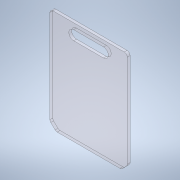
# Autodesk Inventor part: J010355
Saved by Autodesk Inventor 2020.3 (Build 243373000, 373)
## iProperties
RuleStatus: InUse
AfterDocSave0: file://Part Number Cleaner
Created: 2022-05-24
Material: ACRYLIC, CLEAR
Catalog Web Link: https://www.janelia.org/
Vendor: HHMI: JRC - jET
Document SubType Name: Modeling
Designer: arnoldj
Density: 0.66 g/cm^3
Appearance: Polycarbonate (Clear)
Part Number: J010355
Project: COMMON
Description: FB BTM PLATE
LAB/DEPT: COMMON
REQUESTING SCIENTIST: COMMON
SURFACE ROUGHNESS: N/A
DESIGN DEPARTMENT: COMMON
SPECIAL FINISH: NONE
ALTERED ITEM PART NUMBER: N/A
ALTERED ITEM VENDOR: N/A
ALTERED ITEM DESCRIPTION: N/A
Title: Standard
Author: arnoldj
Revision Number: 0
Autodesk Inventor part; units mm, degrees
ref_plane "YZ Plane" through (0, 0, 0) normal (1, 0, 0) x (0, 1, 0)
ref_plane "XZ Plane" through (0, 0, 0) normal (0, 1, 0) x (-1, 0, 0)
ref_plane "XY Plane" through (0, 0, 0) normal (0, 0, 1) x (1, 0, 0)
sketch "Sketch1" plane through (0, 0, 0) normal (0, 0, 1) x (1, 0, 0)
  line L0 (0, 76.454) -> (0, -76.454) projected
  line L1 (-57.4294, 0) -> (57.4294, 0) projected
  line L2 (41.021, -54.61) -> (-41.021, -54.61)
  line L3 (-41.021, -54.61) -> (-41.021, 54.61)
  line L4 (-41.021, 54.61) -> (41.021, 54.61)
  line L5 (41.021, 54.61) -> (41.021, -54.61)
  line L6 (41.021, -54.61) -> (-41.021, 54.61) construction
  line L7 (-41.021, -54.61) -> (41.021, 54.61) construction
  line L8 (15.875, 43.18) -> (-15.875, 43.18) construction
  line L9 (15.875, 48.26) -> (-15.875, 48.26)
  line L10 (-15.875, 38.1) -> (15.875, 38.1)
  arc A0 (15.875, 38.1) -> (15.875, 48.26) centre (15.875, 43.18) ccw
  arc A1 (-15.875, 48.26) -> (-15.875, 38.1) centre (-15.875, 43.18) ccw
  point P0 (0, 0)
  point P1 (0, 43.18)
  dimension "d0" = 82.042
  dimension "d1" = 109.22
  dimension "d4" = 31.75
  dimension "d5" = 6.35
  dimension "d6" = 5.08
  constraints: 20 end point, 4 point on circle, 4 tangent, 3 midpoint, 3 parallel, 2 centre point, 2 perpendicular, 1 horizontal, 1 point on line
  measures "d0" distance of L3.end L4.end
  measures "d1" distance of L2.end L3.end
  measures "d4" distance of L9.start L9.end
  measures "d5" distance between parallel lines of L4 L9
  measures "d6" radius of A1
extrude "Extrusion1" add sketch "Sketch1" along normal blind 2.9972 contours L4 L5 L1 L0 L10 A0 L9 | L0 L9 A1 L10 L1 L3 L4 | L1 L0 L2 L3 | L5 L2 L0 L1
fillet "Fillet1" radius 3.175 2 edges at (-41.021, 54.61, 1.4986) (41.021, 54.61, 1.4986)
chamfer "Chamfer1" distance 6.35 angle 45 2 edges at (41.021, -54.61, 1.4986) (-41.021, -54.61, 1.4986)
fillet "Fillet2" radius 3.175 4 edges at (-41.021, -48.26, 1.4986) (-34.671, -54.61, 1.4986) (34.671, -54.61, 1.4986) (41.021, -48.26, 1.4986)
body "Solid1"
